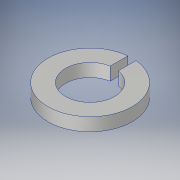
# Autodesk Inventor part: Contre rondelle
Saved by Autodesk Inventor 2017 (Build 210142000, 142)
## iProperties
Company: FABLAB Frenchmakers
Part Number: Contre rondelle
Material: Aluminium
Document SubType Name: Modeling
Designer: FABLAB Frenchmakers
Density: 2.7 g/cm^3
Appearance: Aluminium - Plat(2)
Mass: 0.0285621 g
Surface Area: 0.478611 cm^2
Volume: 0.0105785 cm^3
Project: 1420 Vauban 3D XL
Catalog Web Link: http://frenchmakers.com/
Stock Number: 1420-12-06
Autodesk Inventor part; units mm, degrees
ref_plane "YZ Plane" through (0, 0, 0) normal (1, 0, 0) x (0, 1, 0)
ref_plane "XZ Plane" through (0, 0, 0) normal (0, 1, 0) x (-1, 0, 0)
ref_plane "XY Plane" through (0, 0, 0) normal (0, 0, 1) x (1, 0, 0)
sketch "Esquisse1" plane through (0, 0, 0) normal (0, 0, 1) x (1, 0, 0)
  circle A0 centre (0, 0) radius 1.5
  circle A1 centre (0, 0) radius 2.575
  dimension "d0" = 3
  dimension "d1" = 5.15
  constraints: 2 centre point, 2 coincident
  measures "d0" diameter of A0
  measures "d1" diameter of A1
extrude "Extrusion1" add sketch "Esquisse1" along normal mid plane 0.8
sketch "Esquisse2" plane through (0, 0, 0.4) normal (0, 0, 1) x (1, 0, 0)
  line L0 (-0.25, 0) -> (0.25, 0)
  line L1 (0.25, 0) -> (0.25, 3.075)
  line L2 (0.25, 3.075) -> (-0.25, 3.075)
  line L3 (-0.25, 3.075) -> (-0.25, 0)
  circle A0 centre (0, 0) radius 2.575 projected
  dimension "d4" = 0.5
  dimension "d5" = 0.5
  constraints: 8 end point, 2 parallel, 1 coincident, 1 horizontal, 1 horizontal alignment, 1 midpoint, 1 perpendicular
  measures "d4" distance of L1.end L2.end
  measures "d5" distance edge to line of A0 L2
extrude "Extrusion2" cut sketch "Esquisse2" against normal through all contours L3 A0 L1 L0 | L3 L2 L1 A0 picked at (0.0278, 0.8579)
